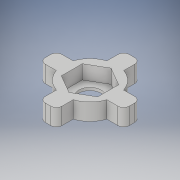
# Autodesk Inventor part: Wing_Nut
Saved by Autodesk Inventor 2019 (Build 230136000, 136)
## iProperties
Created: 2019-10-21
Part Number: Wing_Nut
Material: Generic
Document SubType Name: Modeling
Designer: 19879326
Density: 1 g/cm^3
Appearance: Default
Author: 19879326
Autodesk Inventor part; units mm, degrees
ref_plane "YZ Plane" through (0, 0, 0) normal (1, 0, 0) x (0, 1, 0)
ref_plane "XZ Plane" through (0, 0, 0) normal (0, 1, 0) x (-1, 0, 0)
ref_plane "XY Plane" through (0, 0, 0) normal (0, 0, 1) x (1, 0, 0)
sketch "Sketch1" plane through (0, 0, 0) normal (0, 1, 0) x (-1, 0, 0)
  circle A0 centre (0, 0) radius 9.5
  line L0 (3, 15) -> (-3, 15)
  line L1 (-3, -15) -> (3, -15)
  line L2 (-15, 3) -> (-15, -3)
  line L3 (15, -3) -> (15, 3)
  line L4 (3, -15) -> (3, -9.0139)
  line L5 (3, 9.0139) -> (3, 15)
  line L6 (15, 3) -> (9.0139, 3)
  line L7 (-9.0139, 3) -> (-15, 3)
  line L8 (-3, 15) -> (-3, 9.0139)
  line L9 (-3, -9.0139) -> (-3, -15)
  line L10 (-15, -3) -> (-9.0139, -3)
  line L11 (9.0139, -3) -> (15, -3)
  circle A1 centre (0, 0) radius 4
  point P0 (15, 0)
  point P1 (0, -15)
  point P2 (0, 15)
  point P3 (-15, 0)
  point P4 (9.5, 0)
  dimension "d0" = 19
  dimension "d2" = 6
  dimension "d7" = 5.5
  dimension "d10" = 8
  constraints: 24 end point, 10 parallel, 10 perpendicular, 4 midpoint, 3 horizontal, 3 horizontal alignment, 2 coincident, 2 vertical alignment, 1 centre point, 11 other
  measures "d2" distance of L3.start L3.end
  measures "d7" distance of point (15, 0) point (9.5, 0)
  measures "d10" diameter of A1
extrude "Extrusion1" add sketch "Sketch1" along normal blind 6
fillet "Fillet1" radius 2 8 edges at (3, 3, 15) (-3, 3, 15) (-15, 3, 3) (-15, 3, -3) (-3, 3, -15) (3, 3, -15) (15, 3, -3) (15, 3, 3)
sketch "Sketch2" plane through (0, 6, 0) normal (0, 1, 0) x (1, 0, 0)
  line L0 (-6.5, 3.7528) -> (0, 7.5056)
  line L1 (0, 7.5056) -> (6.5, 3.7528)
  line L2 (6.5, 3.7528) -> (6.5, -3.7528)
  line L3 (6.5, -3.7528) -> (0, -7.5056)
  line L4 (0, -7.5056) -> (-6.5, -3.7528)
  line L5 (-6.5, -3.7528) -> (-6.5, 3.7528)
  line L6 (-15, 1) -> (-15, -1) projected
  point P0 (0, 0)
  point P1 (0, 0)
  dimension "d6" = 13
  constraints: 12 end point, 1 coincident, 1 parallel, 13 other
  measures "d6" distance between parallel lines of L2 L5
extrude "Extrusion2" cut sketch "Sketch2" against normal blind 5
body "Solid1"
